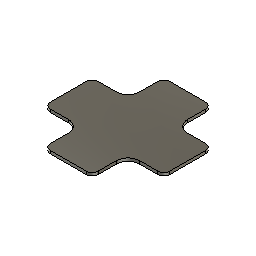
8thLessonFilletComand v2 (Autodesk Fusion 360 design; units mm, degrees)
Autodesk Fusion 360 part; units mm, degrees
sketch "Sketch1" plane through (0, 0, 0) normal (0, 0, 1) x (1, 0, 0)
  line L0 (-10, 20) -> (-10, 60)
  line L1 (90, 60) -> (90, 20)
  line L2 (90, 20) -> (-10, 60) construction
  line L3 (-10, 20) -> (90, 60) construction
  line L4 (60, -10) -> (20, -10)
  line L5 (20, 90) -> (60, 90)
  line L6 (60, -10) -> (20, 90) construction
  line L7 (20, -10) -> (60, 90) construction
  line L8 (-10, 60) -> (10, 60)
  line L9 (70, 60) -> (90, 60)
  line L10 (60, 90) -> (60, 70)
  line L11 (60, 10) -> (60, -10)
  line L12 (90, 20) -> (70, 20)
  line L13 (10, 20) -> (-10, 20)
  line L14 (20, -10) -> (20, 10)
  line L15 (20, 70) -> (20, 90)
  arc A0 (10, 60) -> (20, 70) centre (10, 70) ccw
  arc A1 (60, 70) -> (70, 60) centre (70, 70) ccw
  arc A2 (70, 20) -> (60, 10) centre (70, 10) ccw
  arc A3 (20, 10) -> (10, 20) centre (10, 10) ccw
  point P0 (40, 40)
  point P1 (40, 40)
  dimension "d1" = 100
  dimension "d2" = 40
  dimension "d3" = 40
  dimension "d4" = 100
  dimension "d5" = 10
  dimension "d6" = 10
  dimension "d7" = 10
  dimension "d8" = 10
  constraint horizontal L12
  constraint perpendicular L0 L12
  constraint parallel L8 L12
  constraint parallel L0 L1
  constraint coincident L2 P1
  constraint coincident L3 P1
  constraint horizontal L4
  constraint perpendicular L4 L14
  constraint parallel L4 L5
  constraint parallel L10 L14
  constraint coincident L6 P1
  constraint coincident L7 P1
  constraint coincident P1 P0
  constraint collinear L8 L9
  constraint collinear L10 L11
  constraint collinear L12 L13
  constraint collinear L14 L15
  constraint tangent L15 A0
  constraint tangent L8 A0
  constraint tangent L9 A1
  constraint tangent L10 A1
  constraint tangent L12 A2
  constraint tangent L11 A2
  constraint tangent L13 A3
  constraint tangent L14 A3
  measures "d1" distance of L0.end L1.start
  measures "d2" distance of L0.start L0.end
  measures "d3" distance of L5.start L5.end
  measures "d4" distance of L4.end L5.start
  measures "d5" radius of A0
  measures "d6" radius of A1
  measures "d7" radius of A2
  measures "d8" radius of A3
extrude "Extrude1" add sketch "Sketch1" along normal blind 2.5
fillet "Fillet1" radius 5 1 edges at (60, -10, 1.25)
fillet "Fillet2" radius 5 1 edges at (20, -10, 1.25)
fillet "Fillet3" radius 5 1 edges at (-10, 20, 1.25)
fillet "Fillet4" radius 5 2 edges at (-10, 60, 1.25) (20, 90, 1.25)
fillet "Fillet5" radius 5 2 edges at (60, 90, 1.25) (90, 60, 1.25)
fillet "Fillet6" radius 5 1 edges at (90, 20, 1.25)
